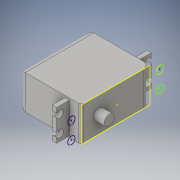
# Autodesk Inventor part: MOTOR
Saved by Autodesk Inventor 2016 (Build 200138000, 138)
## iProperties
Created: 2016-10-04
Part Number: MOTOR
Material: Generic
Document SubType Name: Modeling
Designer: brandn
Density: 1 g/cm^3
Appearance: Default
Author: brandn
Autodesk Inventor part; units mm, degrees
ref_plane "YZ Plane" through (0, 0, 0) normal (1, 0, 0) x (0, 1, 0)
ref_plane "XZ Plane" through (0, 0, 0) normal (0, 1, 0) x (-1, 0, 0)
ref_plane "XY Plane" through (0, 0, 0) normal (0, 0, 1) x (1, 0, 0)
sketch "Sketch1" plane through (0, 0, 0) normal (1, 0, 0) x (0, 1, 0)
  line L0 (10.5023, 21.0047) -> (-9.5637, 21.0047)
  line L1 (-9.5637, 21.0047) -> (-9.5637, -19.2543)
  line L2 (-9.5637, -19.2543) -> (10.5023, -19.2543)
  line L3 (10.5023, -19.2543) -> (10.5023, 21.0047)
  point P0 (0, 0)
  dimension "d0" = 40.259
  dimension "d1" = 20.066
  constraints: 8 end point, 2 parallel, 1 horizontal, 1 perpendicular
  measures "d0" distance of L2.end L0.start
  measures "d1" distance of L0.start L0.end
extrude "Extrusion1" add sketch "Sketch1" along normal blind 35.8902
sketch "Sketch2" plane through (35.8902, 0, 0) normal (1, 0, 0) x (0, 0, -1)
  point P0 (0, 0)
sketch "Sketch3" plane through (35.8902, 0, 0) normal (1, 0, 0) x (0, 0, -1)
  circle A0 centre (-10.6161, 0.6217) radius 2.9238
  line L0 (19.2543, 10.5023) -> (-21.0047, 10.5023) projected
  line L1 (-21.0047, 10.5023) -> (-21.0047, -9.5637) projected
  point P0 (0, 0)
  dimension "d4" = 9.8806
  dimension "d5" = 10.3886
  constraints: 1 centre point
  measures "d4" distance from line of L0 A0.centre
  measures "d5" distance from line of L1 A0.centre
extrude "Extrusion2" add sketch "Sketch3" along normal blind 6.0198
sketch "Sketch4" plane through (0, -9.5637, 21.0047) normal (0, 0, 1) x (1, 0, 0)
  line L0 (29.083, 19.1008) -> (26.6446, 19.1008)
  line L1 (26.6446, 19.1008) -> (26.6446, 0.9652)
  line L2 (26.6446, 0.9652) -> (29.083, 0.9652)
  line L3 (29.083, 0.9652) -> (29.083, 19.1008)
  line L4 (35.8902, 0) -> (35.8902, 20.066) projected
  line L5 (0, 20.066) -> (0, 0) projected
  line L6 (0, 20.066) -> (35.8902, 20.066) projected
  line L7 (0, 0) -> (35.8902, 0) projected
  point P0 (0, 9.5637)
  dimension "d8" = 6.8072
  dimension "d9" = 26.6446
  dimension "d12" = 35.8902
  dimension "d13" = 0.9652
  dimension "d14" = 0.9652
  constraints: 8 end point, 2 parallel, 1 horizontal, 1 perpendicular
  measures "d8" distance between parallel lines of L4 L3
  measures "d9" distance between parallel lines of L5 L1
  measures "d12" distance between parallel lines of L5 L4
  measures "d13" distance between parallel lines of L6 L0
  measures "d14" distance between parallel lines of L7 L2
extrude "Extrusion3" add sketch "Sketch4" along normal blind 7.5692 contours L3 L2 L1 L0
sketch "Sketch5" plane through (29.083, -8.5985, 21.0047) normal (1, 0, 0) x (0, 0, -1)
  circle A0 centre (-5.766, 14.0716) radius 2.1717
  circle A1 centre (-5.766, 4.064) radius 2.1717
  line L0 (0, 0) -> (-7.5692, 0) projected
  line L1 (0, 18.1356) -> (-7.5692, 18.1356) projected
  point P0 (21.0047, 8.5985)
  dimension "d17" = 4.3434
  dimension "d18" = 4.3434
  dimension "d20" = 4.064
  dimension "d22" = 4.064
  constraints: 2 centre point
  measures "d17" diameter of A0
  measures "d18" diameter of A1
  measures "d20" distance from line of L0 A1.centre
  measures "d22" distance from line of L1 A0.centre
sketch "Sketch6" plane through (29.083, -8.5985, 21.0047) normal (1, 0, 0) x (0, 0, -1)
  point P0 (21.0047, 8.5985)
extrude "Extrusion4" cut sketch "Sketch5" against normal blind 2.4384
sketch "Sketch7" plane through (0, 10.5023, -19.2543) normal (0, 0, -1) x (1, 0, 0)
  line L0 (29.083, 19.1008) -> (26.6446, 19.1008)
  line L1 (26.6446, 19.1008) -> (26.6446, 0.9652)
  line L2 (26.6446, 0.9652) -> (29.083, 0.9652)
  line L3 (29.083, 0.9652) -> (29.083, 19.1008)
  line L4 (35.8902, 0) -> (35.8902, 20.066)
  line L5 (0, 20.066) -> (0, 0)
  line L6 (0, 20.066) -> (35.8902, 20.066)
  line L7 (0, 0) -> (35.8902, 0)
  point P0 (0, 9.5637)
  dimension "d25" = 6.8072
  dimension "d27" = 26.6446
  dimension "d39" = 35.8902
  dimension "d28" = 0.9652
  dimension "d26" = 0.9652
  constraints: 16 end point, 2 parallel, 1 horizontal, 1 perpendicular
  measures "d25" distance between parallel lines of L4 L3
  measures "d27" distance between parallel lines of L5 L1
  measures "d39" distance between parallel lines of L5 L4
  measures "d28" distance between parallel lines of L6 L0
  measures "d26" distance between parallel lines of L7 L2
extrude "Extrusion5" add sketch "Sketch7" along normal blind 7.5692 contours L3 L2 L1 L0
sketch "Sketch8" plane through (29.083, 9.5371, -19.2543) normal (1, 0, 0) x (0, 0, 1)
  circle A0 centre (-5.766, 14.0716) radius 2.1717
  circle A1 centre (-5.766, 4.064) radius 2.1717
  line L0 (0, 0) -> (-7.5692, 0) projected
  line L1 (0, 18.1356) -> (-7.5692, 18.1356) projected
  point P0 (21.0047, 8.5985)
  dimension "d34" = 4.3434
  dimension "d32" = 4.3434
  dimension "d33" = 4.064
  dimension "d35" = 4.064
  constraints: 2 centre point
  measures "d34" diameter of A0
  measures "d32" diameter of A1
  measures "d33" distance from line of L0 A1.centre
  measures "d35" distance from line of L1 A0.centre
extrude "Extrusion6" cut sketch "Sketch8" against normal blind 2.4384
fillet "Fillet1" radius 3.175 4 edges at (0, 10.5023, 0.8752) (0, -9.5637, 0.8752) (0, 0.4693, -19.2543) (0, 0.4693, 21.0047)
fillet "Fillet2" radius 1.5875 1 edges at (35.8902, 0.4693, 21.0047)
fillet "Fillet3" radius 3.81 1 edges at (35.8902, 0.4693, -19.2543)
sketch "Sketch9" plane through (35.8902, 0, 0) normal (1, 0, 0) x (0, 0, -1)
  line L0 (-19.4172, -9.5637) -> (15.4443, -9.5637) projected
  line L1 (15.4443, 10.5023) -> (-19.4172, 10.5023) projected
  line L2 (-21.0047, 10.5023) -> (-21.0047, -9.5637) projected
  line L3 (19.2543, -9.5637) -> (19.2543, 10.5023) projected
  line L4 (19.2543, -9.5637) -> (15.4443, -9.5637) projected
  line L5 (15.4443, 10.5023) -> (19.2543, 10.5023) projected
  line L6 (-21.0047, 10.5023) -> (-19.4172, 10.5023) projected
  line L7 (-19.4172, -9.5637) -> (-21.0047, -9.5637) projected
  arc A0 (-28.5739, 4.2629) -> (-28.5739, 6.6834) centre (-26.7707, 5.4731) ccw projected
  circle A1 centre (-26.7707, 5.4731) radius 2.1717
  arc A2 (-28.5739, -5.7447) -> (-28.5739, -3.3242) centre (-26.7707, -4.5345) ccw projected
  circle A3 centre (-26.7707, -4.5345) radius 2.1717
  arc A4 (26.8235, 6.6834) -> (26.8235, 4.2629) centre (25.0203, 5.4731) ccw projected
  circle A5 centre (25.0203, 5.4731) radius 2.1717
  circle A6 centre (25.0203, -4.5345) radius 2.1717
  point P0 (0, 0)
  constraints: 3 coincident, 2 centre point, 6 other
body "Solid1"
